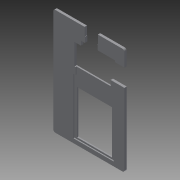
# Autodesk Inventor part: DisplayMid2
Saved by Autodesk Inventor 2014 SP1 (Build 180222100, 222)
## iProperties
Created: 2014-03-24
Part Number: DisplayMid2
Material: Generic
Document SubType Name: Modeling
Designer: patrigg
Density: 1 g/cm^3
Appearance: Default
Author: patrigg
Autodesk Inventor part; units mm, degrees
ref_plane "YZ Plane" through (0, 0, 0) normal (1, 0, 0) x (0, 1, 0)
ref_plane "XZ Plane" through (0, 0, 0) normal (0, 1, 0) x (-1, 0, 0)
sketch "Sketch2" plane through (0, 0, 0) normal (0, 1, 0) x (-1, 0, 0)
  line L0 (-33.5, -50) -> (33.5, -50)
  line L1 (33.5, -50) -> (33.5, 50)
  line L2 (33.5, 50) -> (-33.5, 50)
  line L3 (-33.5, 50) -> (-33.5, -50)
  line L4 (-33.5, -50) -> (33.5, 50) construction
  line L5 (33.5, -50) -> (-33.5, 50) construction
  point P0 (0, 0)
  dimension "d0" = 67
  dimension "d1" = 100
  constraints: 12 end point, 2 midpoint, 2 parallel, 1 horizontal, 1 perpendicular
  measures "d0" distance of L2.end L1.end
  measures "d1" distance of L1.end L0.end
extrude "Extrusion1" add sketch "Sketch2" along normal blind 4
sketch "Sketch3" plane through (0, 4, 0) normal (0, 1, 0) x (1, 0, 0)
  line L0 (33.5, 50) -> (-33.5, 50) projected
  line L1 (-14.5, -6.5) -> (23.5, -6.5)
  line L2 (23.5, -6.5) -> (23.5, 46)
  line L3 (23.5, 46) -> (-14.5, 46)
  line L4 (-14.5, 46) -> (-14.5, -6.5)
  line L5 (-14.5, -6.5) -> (23.5, 46) construction
  line L6 (23.5, -6.5) -> (-14.5, 46) construction
  line L7 (33.5, -50) -> (33.5, 50) projected
  point P0 (0, 0)
  point P1 (4.5, 19.75)
  dimension "d4" = 38
  dimension "d5" = 52.5
  dimension "d6" = 4
  dimension "d104" = 10
  constraints: 12 end point, 2 midpoint, 2 parallel, 1 horizontal, 1 perpendicular
  measures "d4" distance of L3.end L2.end
  measures "d5" distance of L2.end L1.end
  measures "d6" distance between parallel lines of L0 L3
  measures "d104" distance between parallel lines of L7 L2
extrude "Extrusion2" cut sketch "Sketch3" against normal blind 2.75
sketch "Sketch4" plane through (0, 1.25, 0) normal (0, 1, 0) x (1, 0, 0)
  line L0 (23.5, -6.5) -> (-14.5, -6.5) projected
  line L1 (23.5, 46) -> (23.5, -6.5) projected
  line L2 (-14.5, 46) -> (23.5, 46) projected
  line L3 (-14.5, -6.5) -> (-14.5, 46) projected
  line L4 (-12, 44.5) -> (21, 44.5)
  line L5 (21, 44.5) -> (21, 3.5)
  line L6 (21, 3.5) -> (-12, 3.5)
  line L7 (-12, 3.5) -> (-12, 44.5)
  line L8 (-12, 44.5) -> (21, 3.5) construction
  line L9 (21, 44.5) -> (-12, 3.5) construction
  point P0 (0, 0)
  point P1 (4.5, 24)
  dimension "d9" = 10
  dimension "d10" = 1.5
  dimension "d11" = 2.5
  dimension "d12" = 2.5
  constraints: 12 end point, 2 midpoint, 2 parallel, 1 horizontal, 1 perpendicular
  measures "d9" distance between parallel lines of L0 L6
  measures "d10" distance between parallel lines of L2 L4
  measures "d11" distance between parallel lines of L1 L5
  measures "d12" distance between parallel lines of L3 L7
extrude "Extrusion3" cut sketch "Sketch4" against normal blind 2.5 contours L4 L5 L6 L7
sketch "Sketch5" plane through (0, 4, 0) normal (0, 1, 0) x (1, 0, 0)
  line L0 (23.5, 46) -> (23.5, -6.5) projected
  line L1 (23.5, -6.5) -> (-14.5, -6.5) projected
  line L2 (-14.5, -6.5) -> (-14.5, 46) projected
  line L3 (-12.5, -13) -> (-12.5, -6.5)
  line L4 (21.5, -13) -> (21.5, -6.5)
  line L5 (33.5, 50) -> (-33.5, 50) projected
  line L6 (-12.5, -13) -> (21.5, -13)
  point P0 (0, 0)
  dimension "d18" = 2
  dimension "d19" = 2
  dimension "d112" = 6.5
  constraints: 6 end point, 2 perpendicular, 2 point on line, 1 parallel
  measures "d18" distance between parallel lines of L3 L2
  measures "d19" distance between parallel lines of L0 L4
  measures "d112" distance between parallel lines of L1 L6
extrude "Extrusion4" cut sketch "Sketch5" against normal blind 0.25
sketch "Sketch12" plane through (0, 4, 0) normal (0, 1, 0) x (1, 0, 0)
  line L0 (21.5, -13) -> (-12.5, -13) projected
  line L1 (-13.5, -37) -> (24.5, -37)
  line L2 (24.5, -37) -> (24.5, -13)
  line L3 (24.5, -13) -> (-13.5, -13)
  line L4 (-13.5, -13) -> (-13.5, -37)
  line L5 (-13.5, -37) -> (24.5, -13) construction
  line L6 (24.5, -37) -> (-13.5, -13) construction
  line L7 (23.5, 46) -> (23.5, -6.5) projected
  point P0 (0, 0)
  point P1 (5.5, -25)
  point P2 (5.5, -25)
  dimension "d58" = 38
  dimension "d59" = 24
  dimension "d105" = 1
  constraints: 12 end point, 3 midpoint, 2 parallel, 1 collinear, 1 horizontal, 1 perpendicular
  measures "d58" distance of L3.end L2.end
  measures "d59" distance of L2.end L1.end
  measures "d105" distance between parallel lines of L7 L2
extrude "Extrusion10" cut sketch "Sketch12" against normal blind 4
sketch "Sketch13" plane through (24.5, 4, 13) normal (-1, 0, 0) x (0, 0, 1)
  line L0 (0, 0) -> (24, 0) projected
  line L1 (0, 0) -> (0, -4) projected
  line L2 (24, -4) -> (0, -4) projected
  line L3 (6, 0) -> (6, -4)
  line L4 (0, -2.2) -> (6, -2.2)
  point P0 (-13, -4)
  dimension "d67" = 6
  dimension "d74" = 1.8
  constraints: 4 end point, 4 point on line, 2 perpendicular
  measures "d67" distance between parallel lines of L3 L1
  measures "d74" distance between parallel lines of L2 L4
sketch "Sketch14" plane through (-13.5, 4, 37) normal (1, 0, 0) x (0, 0, -1)
  line L0 (0, 0) -> (24, 0) projected
  line L1 (0, 0) -> (0, -4)
  line L2 (4.0418, -2.2) -> (4.0418, 0)
  line L3 (24, -4) -> (0, -4) projected
  line L4 (0, -2.2) -> (4.0418, -2.2)
  point P0 (37, -4)
  point P1 (0, -2)
  dimension "d79" = 1.8
  constraints: 6 end point, 2 perpendicular, 2 point on line, 1 midpoint
  measures "d79" distance between parallel lines of L3 L4
extrude "Extrusion13" add sketch "Sketch13" along normal blind 4 contours L0 L3 L4 L1
extrude "Extrusion14" add sketch "Sketch14" along normal blind 6
sketch "Sketch16" plane through (0, 3.75, 0) normal (0, 1, 0) x (1, 0, 0)
  line L0 (-12.5, -13) -> (-12.5, -6.5) projected
  line L1 (20.5, -13) -> (-12.5, -13) projected
  line L2 (21.5, -13) -> (20.5, -13) projected
  line L3 (21.5, -6.5) -> (21.5, -13) projected
  line L4 (-12.5, -6.5) -> (21.5, -6.5) projected
  point P0 (0, 0)
extrude "Extrusion15" cut sketch "Sketch16" against normal up to next
sketch "Sketch17" plane through (21.5, 4, 6.5) normal (-1, 0, 0) x (0, 0, 1)
  line L0 (0, -2.75) -> (0, -4) projected
  line L1 (6.5, -4) -> (0, -4) projected
  line L2 (6.5, -2.2) -> (6.5, -4) projected
  line L3 (6.5, 0) -> (6.5, -2.2) projected
  line L4 (0, -2.75) -> (-1.7339, -2.75) construction
  line L5 (5.5, -4) -> (7.1842, -4) construction
  line L6 (0, -2.75) -> (5.5, -4) construction
  arc A0 (2.3486, -3.3) -> (0, -2.75) centre (0, -8.0397) ccw
  line L7 (0, -2.75) -> (0, 0) projected
  line L8 (2.3486, -4) -> (2.3486, -3.3)
  line L9 (0, 0) -> (6.5, 0) projected
  line L10 (0, -1.25) -> (6.5, -1.25)
  point P0 (-6.5, -4)
  dimension "d82" = 1
  dimension "d86" = 0.7
  dimension "d95" = 1.25
  constraints: 10 end point, 4 point on line, 2 parallel, 2 perpendicular, 2 point on circle, 1 centre point, 1 tangent
  measures "d82" distance from line of L2 L5.start
  measures "d86" distance of L8.start L8.end
  measures "d95" distance between parallel lines of L10 L9
extrude "Extrusion16" add sketch "Sketch17" along normal up to next contours A0 L8 L1 L0 | L7 L9 L3 L10
fillet "Fillet5" radius 1 1 edges at (4.5, 0.7, 8.8486)
sketch "Sketch18" plane through (23.5, 4, -46) normal (-1, 0, 0) x (0, 0, 1)
  line L0 (0, 0) -> (52.5, 0) projected
  line L1 (0, 0) -> (0, -2.75) projected
  line L2 (52.5, 0) -> (52.5, -2.75) projected
  line L3 (0, -1.25) -> (52.5, -1.25)
  line L4 (1.5, -2.75) -> (1.5, -4) projected
  line L5 (42.5, -2.75) -> (42.5, -4) projected
  dimension "d88" = 1.25
  constraints: 2 end point, 2 point on line, 1 perpendicular
  measures "d88" distance between parallel lines of L3 L0
extrude "Extrusion17" add sketch "Sketch18" along normal up to next
sketch "Sketch21" plane through (0, 4, 0) normal (0, 1, 0) x (1, 0, 0)
  line L0 (21, 44.5) -> (-12, 44.5) projected
  line L1 (21, 3.5) -> (21, 44.5) projected
  line L2 (-12, 44.5) -> (-12, 3.5) projected
  line L3 (-12, 3.5) -> (21, 3.5) projected
  point P0 (0, 0)
extrude "Extrusion19" cut sketch "Sketch21" against normal up to next
sketch "Sketch23" plane through (0, 4, 0) normal (0, 1, 0) x (1, 0, 0)
  line L0 (24.5, -19) -> (24.5, -37) projected
  line L1 (24.5, -37) -> (-7.5, -37) projected
  line L2 (33.5, -50) -> (33.5, 50) projected
  line L3 (24.5, -19) -> (33.5, -19)
  line L4 (24.5, -35.5) -> (33.5, -35.5)
  point P0 (0, 0)
  dimension "d106" = 1.5
  constraints: 4 end point, 3 point on line, 1 parallel, 1 perpendicular
  measures "d106" distance between parallel lines of L4 L1
extrude "Extrusion21" cut sketch "Sketch23" against normal blind 2.2
sketch "Sketch25" plane through (0, 4, 0) normal (0, 1, 0) x (1, 0, 0)
  line L0 (-33.5, -50) -> (33.5, -50) projected
  line L1 (24.5, -35.5) -> (24.5, -37) projected
  line L2 (-4, -42) -> (8.5, -42)
  line L3 (8.5, -42) -> (8.5, -50)
  line L4 (8.5, -50) -> (-4, -50)
  line L5 (-4, -50) -> (-4, -42)
  line L6 (-4, -42) -> (8.5, -50) construction
  line L7 (8.5, -42) -> (-4, -50) construction
  line L8 (-3.75, -37) -> (8.25, -37)
  line L9 (8.25, -37) -> (8.25, -42)
  line L10 (8.25, -42) -> (-3.75, -42)
  line L11 (-3.75, -42) -> (-3.75, -37)
  line L12 (-3.75, -37) -> (8.25, -42) construction
  line L13 (8.25, -37) -> (-3.75, -42) construction
  line L14 (24.5, -37) -> (-7.5, -37) projected
  point P0 (0, 0)
  point P1 (2.25, -46)
  point P2 (2.25, -39.5)
  point P3 (2.25, -39.5)
  point P4 (2.25, -46)
  dimension "d113" = 12.5
  dimension "d114" = 8
  dimension "d116" = 12
  dimension "d117" = 16
  constraints: 24 end point, 6 midpoint, 4 parallel, 2 collinear, 2 horizontal, 2 perpendicular, 1 point on line, 1 vertical alignment
  measures "d113" distance of L3.end L4.end
  measures "d114" distance of L2.end L3.end
  measures "d116" distance between parallel lines of L9 L11
  measures "d117" distance between parallel lines of L3 L1
extrude "Extrusion22" cut sketch "Sketch25" against normal blind 2.5
fillet "Fillet6" radius 2 4 edges at (33.5, 2, 50) (-33.5, 2, 50) (33.5, 2, -50) (-33.5, 2, -50)
ref_plane "Work Plane1" through (33.5, 1.8, 19) normal (0, 1, 0) x (1, 0, 0)
split body "Split1" result two bodies by plane through (33.5, 1.8, 19) normal (0, 1, 0) first body at (-26.8333, 3.5, 4.3333) (21.5, 3.5, 45.6667)
body "Solid2"
body "Solid3"
